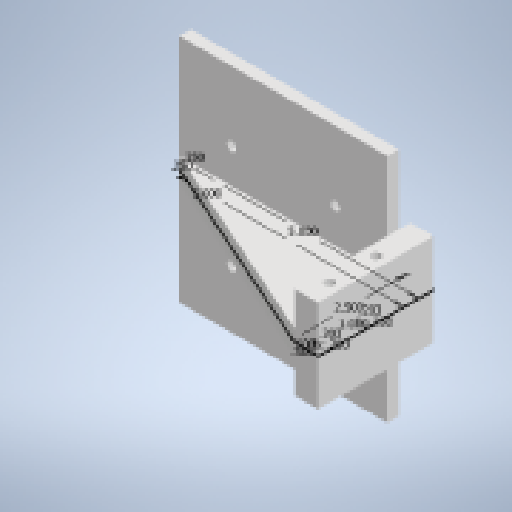
# Autodesk Inventor part: Finger
Saved by Autodesk Inventor 2023 (Build 270158000, 158)
## iProperties
Created: 2023-01-25
Part Number: Finger
Material: Generic
Document SubType Name: Modeling
Designer: Gabriel - T3 CAD
Density: 1 g/cm^3
Appearance: Default
Mass: 260.383 g
Surface Area: 499.728 cm^2
Volume: 260.383 cm^3
Author: Gabriel - T3 CAD
Autodesk Inventor part; units mm, degrees
ref_plane "YZ Plane" through (0, 0, 0) normal (1, 0, 0) x (0, 1, 0)
ref_plane "XZ Plane" through (0, 0, 0) normal (0, 1, 0) x (-1, 0, 0)
ref_plane "XY Plane" through (0, 0, 0) normal (0, 0, 1) x (1, 0, 0)
sketch "Sketch1" plane through (0, 0, 0) normal (0, 1, 0) x (-1, 0, 0)
  line L0 (0, 0) -> (12.7, 0)
  line L1 (12.7, 0) -> (12.7, 63.5)
  line L2 (12.7, 63.5) -> (0, 63.5)
  line L3 (0, 63.5) -> (0, 0)
  line L4 (0, 0) -> (127, 0)
  line L5 (127, 0) -> (127, 6.35)
  line L6 (127, 6.35) -> (0, 6.35)
  line L7 (0, 6.35) -> (0, 0)
  circle A0 centre (6.35, 50.8) radius 2.5797
  circle A1 centre (6.35, 25.4) radius 2.5797
  line L8 (0, 6.35) -> (0, 12.7)
  line L9 (0, 12.7) -> (127, 12.7)
  line L10 (127, 12.7) -> (127, 6.35)
  line L11 (127, 6.35) -> (0, 6.35)
  line L12 (127, 12.7) -> (12.7, 63.5)
  point P0 (12.7, 6.35)
  point P1 (12.7, 0)
  point P2 (12.7, 12.7)
  dimension "d0" = 12.7
  dimension "d1" = 63.5
  dimension "d2" = 127
  dimension "d3" = 6.35
  dimension "d4" = 25.4
  dimension "d5" = 6.35
  dimension "d6" = 6.35
  dimension "d7" = 12.7
  dimension "d8" = 5.1594
  dimension "d9" = 5.1594
  dimension "d24" = 6.35
  dimension "d25" = 127
  constraints: 26 end point, 6 parallel, 3 perpendicular, 2 centre point, 2 horizontal, 1 point on line
  measures "d0" distance of L2.end L1.end
  measures "d1" distance of L1.end L0.end
  measures "d2" distance of L6.end L5.end
  measures "d3" distance of L5.end L4.end
  measures "d4" distance of A1.centre A0.centre
  measures "d5" distance from line of L3 A0.centre
  measures "d6" distance from line of L3 A1.centre
  measures "d7" distance from line of L2 A0.centre
  measures "d8" diameter of A0
  measures "d9" diameter of A1
  measures "d24" distance of L9.end L10.end
  measures "d25" distance of L8.end L9.end
extrude "Extrusion1" add sketch "Sketch1" along normal mid plane 50.8 contours L3 L6 L1 L0 | L3 L9 L1 L6 | L3 L2 L1 L9
extrude "Extrusion2" add sketch "Sketch1" along normal mid plane 127 contours L1 L9 L10 L6
extrude "Extrusion5" add sketch "Sketch1" along normal mid plane 12.7 contours L1 L12 L9
sketch "Sketch3" plane through (-12.7, 63.5, 6.35) normal (0, 0, -1) x (-1, 0, 0)
  circle A0 centre (85.725, -95.25) radius 2.5797
  line L0 (114.3, -127) -> (114.3, 0) projected
  line L1 (114.3, -127) -> (0, -127) projected
  circle A1 centre (28.575, -95.25) radius 2.5797
  circle A2 centre (85.725, -38.1) radius 2.5797
  circle A3 centre (28.575, -38.1) radius 2.5797
  point P0 (-12.7, -63.5)
  dimension "d26" = 5.1594
  dimension "d27" = 28.575
  dimension "d28" = 31.75
  dimension "d31" = 57.15
  dimension "d34" = 57.15
  constraints: 4 centre point, 1 horizontal, 1 vertical, 6 other
  measures "d26" diameter of A0
  measures "d27" distance from line of L0 A0.centre
  measures "d28" distance from line of L1 A0.centre
  measures "d31" distance of A0.centre A1.centre
  measures "d34" distance of A0.centre A2.centre
extrude "Extrusion6" cut sketch "Sketch3" against normal blind 12.7
equation "\"d5\" = 0.5 * d0"
equation "\"d6\" = d5"
equation "\"d31\" = 2 * d27"
equation "\"d34\" = 2 * d27"
body "Solid1"
